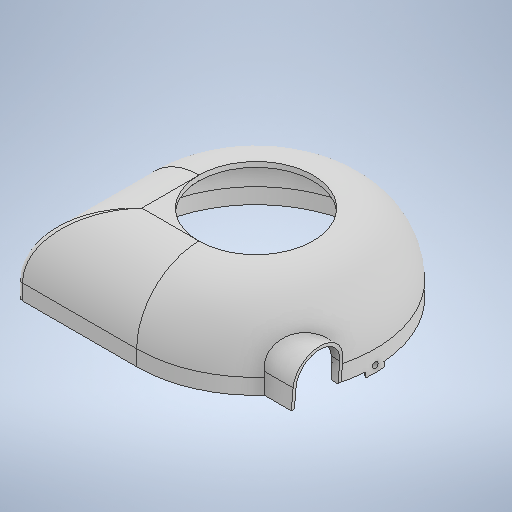
# Autodesk Inventor part: Cylinder Housing_cap_3
Saved by Autodesk Inventor 2025 (Build 290162000, 162)
## iProperties
Created: 2025-10-06
Part Number: Cylinder Housing_cap_3
Material: Generic
Document SubType Name: Modeling
Designer: mumin
Density: 1 g/cm^3
Appearance: Default
Author: mumin
Autodesk Inventor part; units mm, degrees
ref_plane "XZ Plane" through (0, 0, 0) normal (0, 1, 0) x (-1, 0, 0)
ref_plane "XY Plane" through (0, 0, 0) normal (0, 0, 1) x (1, 0, 0)
sketch "Sketch1" plane through (0, 0, 0) normal (0, 1, 0) x (-1, 0, 0)
  arc A0 (0, 115) -> (115, 0) centre (0, 0) ccw
  line L0 (115, 0) -> (115, 110)
  line L1 (110, 115) -> (0, 115)
  arc A1 (115, 110) -> (110, 115) centre (110, 110) ccw
  dimension "d0" = 230
  dimension "d1" = 5
  constraints: 4 end point, 4 point on circle, 2 centre point, 2 tangent, 1 coincident
  measures "d0" diameter of A0
  measures "d1" radius of A1
extrude "Base Shape & Wall" add sketch "Sketch1" along normal blind 75
fillet "Curved Edge" radius 60 4 edges at (81.3173, 75, -81.3173) (-115, 75, 55) (-113.5355, 75, 113.5355) (-55, 75, 115)
shell "Shell" thickness 4.9 removed faces 1 at (-52.6749, 0, -2.0856)
sketch "Sketch2" plane through (0, 75, 0) normal (0, 1, 0) x (1, 0, 0)
  point P0 (0, 0)
  point P1 (0, 0)
  constraints: 1 coincident
hole "Cylinder Hole" at (0, 75, 0) direction (0, -1, 0) diameter 110 end through all
sketch "Sketch3" plane through (0, 0, 0) normal (0, -1, 0) x (1, 0, 0)
  arc A0 (-115, 0) -> (0, 115) centre (0, 0) ccw projected
  line L0 (0, 55) -> (0, 110.1) projected
  line L1 (-110.1, 0) -> (-55, 0) projected
  arc A1 (-110.1, 0) -> (0, 110.1) centre (0, 0) ccw projected
  line L2 (114.6551, 8.9) -> (109.9418, 5.9)
  line L3 (109.9418, -5.9) -> (114.6551, -8.9)
  line L4 (-199.1076, 0) -> (222.9249, 0) projected
  arc A2 (-55, 0) -> (0, 55) centre (0, 0) ccw projected
  dimension "d13" = 5.9
  dimension "d14" = 8.9
  constraints: 4 end point, 4 point on circle, 2 symmetric about line
  measures "d13" distance from line of L4 L2.end
  measures "d14" distance from line of L4 L2.start
extrude "Front Tab" add sketch "Sketch3" along normal blind 5 contours L3 A1 L4 A0 | L4 A1 L2 A0 picked at (113.1479, -6.9122)
sketch "Sketch4" plane through (0, 0, 0) normal (1, 0, 0) x (0, 1, 0)
  line L0 (0, 0) -> (15, 0) projected
  circle A0 centre (1.5, 0) radius 2.75
  line L1 (-5, 8.9) -> (-5, -8.9) projected
  dimension "d17" = 5.5
  dimension "d18" = 6.5
  constraints: 1 centre point, 1 point on line
  measures "d17" diameter of A0
  measures "d18" distance from line of L1 A0.centre
extrude "Bolt Hole" cut sketch "Sketch4" along normal through all
sketch "Sketch5" plane through (0, 0, 0) normal (0, 0, 1) x (1, 0, 0)
  line L0 (115, 15) -> (-115, 15) projected
  line L1 (110.1, 15) -> (-110.1, 15) projected
  line L2 (-110.1, 0) -> (-110.1, 15) projected
  line L3 (-110.1, 0) -> (-110.1, 15)
  line L4 (-110.1, 15) -> (-112.6, 15)
  line L5 (-110.1, 0) -> (-112.6, 15)
  line L6 (-110.1, 0) -> (-108.0437, 0)
  line L7 (-108.0437, 0) -> (-108.0437, 15)
  point P0 (0, 0)
  point P1 (0, 15)
  dimension "d22" = 2.5
  constraints: 10 end point, 2 point on line, 1 collinear, 1 horizontal, 1 perpendicular
  measures "d22" distance of L4.end L1.end
extrude "Hinge Tab Recess" cut sketch "Sketch5" along normal mid plane 15
sketch "Sketch6" plane through (0, 0, 0) normal (1, 0, 0) x (0, 1, 0)
  arc A0 (20, 32.226) -> (20, 74.226) centre (20, 53.226) ccw
  line L0 (0, 8.9) -> (0, 115) projected
  line L1 (20, 74.226) -> (0, 74.226)
  line L2 (0, 74.226) -> (0, 32.226)
  line L3 (0, 32.226) -> (20, 32.226)
  point P0 (0, 0)
  dimension "d25" = 42
  dimension "d26" = 53.226
  dimension "d27" = 20
  constraints: 6 end point, 2 point on circle, 1 centre point, 1 horizontal, 1 parallel, 1 perpendicular, 1 point on line
  measures "d25" diameter of A0
  measures "d26" vertical distance of point (0, 0) A0.centre
  measures "d27" distance from line of L0 A0.centre
extrude "Extrusion5" cut sketch "Sketch6" along normal through all
ref_plane "Work Plane1" through (115, 0, 0) normal (1, 0, 0) x (0, 1, 0)
sketch "Sketch8" plane through (115, 0, 0) normal (1, 0, 0) x (0, 1, 0)
  spline S0 degree 5 poles (20, 74.226) (21.7452, 74.226) (23.5079, 74.045) (25.2552, 73.6747) (26.9529, 73.1202) (29.9438, 71.784) (31.2609, 71.0468) (32.4954, 70.2012) (33.6326, 69.2644) (35.8574, 67.094) (36.9093, 65.8358) (37.811, 64.5157) (38.5629, 63.1597) (39.9244, 60.1101) (40.4634, 58.4091) (40.8112, 56.7153) (40.9848, 55.0472) (41.0281, 50.1315) (40.4151, 46.9848) (39.2704, 44.0382) (37.5933, 41.2886) (34.2813, 37.7546) (33.1162, 36.7127) (31.8193, 35.7519) (30.3873, 34.8935) (28.01, 33.793) (27.1625, 33.4531) (26.2801, 33.1539) (25.3653, 32.9001) (23.9884, 32.6034) (23.5482, 32.5207) (23.1027, 32.4491) (22.6524, 32.3892) (21.7638, 32.2956) (21.3262, 32.261) (20.8833, 32.2376) (20.4431, 32.226) (20, 32.226) knots 0 0 0 0 0 0 0.115277 0.115277 0.115277 0.115277 0.213785 0.213785 0.213785 0.213785 0.327655 0.327655 0.327655 0.327655 0.466839 0.466839 0.466839 0.466839 0.745876 0.745876 0.745876 0.745876 0.873844 0.873844 0.873844 0.873844 0.940211 0.940211 0.940211 0.940211 0.970786 0.970786 0.970786 0.970786 1 1 1 1 1 1 projected
  line L0 (15, 74.226) -> (20, 74.226) projected
  line L1 (0, 74.226) -> (15, 74.226) projected
  line L2 (20, 32.226) -> (15, 32.226) projected
  line L3 (15, 32.226) -> (0, 32.226) projected
  line L4 (0, 29.226) -> (15, 29.226)
  line L5 (15, 29.226) -> (20, 29.226)
  line L6 (20, 77.226) -> (15, 77.226)
  line L7 (15, 77.226) -> (0, 77.226)
  line L8 (0, 77.226) -> (0, 74.226)
  line L9 (0, 0) -> (0, 110) projected
  line L10 (0, 32.226) -> (0, 29.226)
  spline S1 degree 5 poles (20, 29.226) (24.9777, 29.2263) (29.9563, 30.5154) (34.4863, 33.1008) (41.4168, 40.0057) (44.3283, 49.2848) (44.6352, 53.9403) (42.8551, 64.1602) (36.1874, 72.3028) (31.2207, 75.5896) (25.6093, 77.2254) (20, 77.226) knots 0 0 0 0 0 0 0.330105 0.330105 0.330105 0.628 0.628 0.628 1 1 1 1 1 1
  dimension "d38" = 3
  constraints: 12 end point, 2 collinear, 2 parallel, 2 vertical alignment, 4 other
extrude "LV Hood" add sketch "Sketch8" against normal up to surface contours L0 L1 L8 L7 L6 S1 L5 L4 L9 L3 L2 S0
sketch "Sketch9" plane through (115, 0, 77.226) normal (0, 0, 1) x (1, 0, 0)
  line L0 (-3.7757, 15) -> (-3.7757, 0) projected
  line L1 (0, 20) -> (-3.9915, 20) projected
  line L2 (0, 0) -> (0, 20) projected
  line L3 (0, 0) -> (-3.7757, 0) projected
  line L4 (0, 20) -> (0, 44) projected
  line L5 (-3.7757, 0) -> (0, 44)
  line L6 (0, 44) -> (0, 0)
  point P0 (-115, 0)
  constraints: 4 end point, 1 collinear, 1 other
extrude "Hood Slant Cut" cut sketch "Sketch9" against normal up to surface (48 mm away)
body "Solid1"
